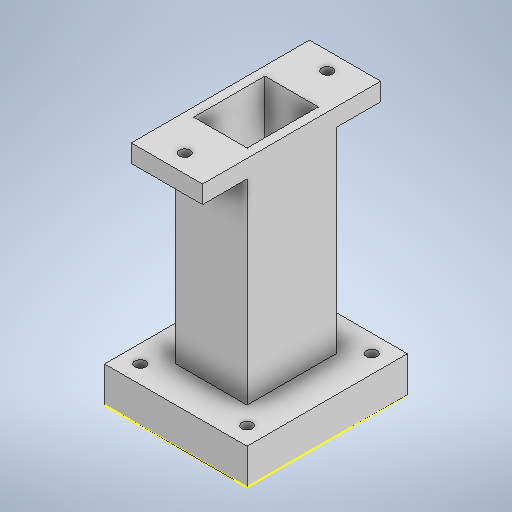
# Autodesk Inventor part: select support V3
Saved by Autodesk Inventor 2025.3 (Build 293356000, 356)
## iProperties
Created: 2026-05-01
Part Number: select support V3
Material: Generic
Document SubType Name: Modeling
Designer: kamal
Density: 1 g/cm^3
Appearance: Default
Author: kamal
## iProperties of the stored document select support V3_3DPrint.ipt
Created: 2026-05-01
Part Number: select support V3_3DPrint
Material: Generic
Document SubType Name: Modeling
Designer: kamal
Density: 1 g/cm^3
Appearance: Default
Author: kamal
Autodesk Inventor part; units mm, degrees
ref_plane "YZ Plane" through (0, 0, 0) normal (1, 0, 0) x (0, 1, 0)
ref_plane "XZ Plane" through (0, 0, 0) normal (0, 1, 0) x (-1, 0, 0)
ref_plane "XY Plane" through (0, 0, 0) normal (0, 0, 1) x (1, 0, 0)
sketch "Sketch1" plane through (0, 0, 0) normal (0, 1, 0) x (-1, 0, 0)
  line L0 (0, 0) -> (5, 0)
  line L1 (5, 0) -> (5, -10)
  line L2 (5, -10) -> (0, -10)
  line L3 (0, -10) -> (0, 0)
  line L4 (-7.5, 20) -> (12.5, 20)
  line L5 (12.5, 20) -> (12.5, -30)
  line L6 (12.5, -30) -> (-7.5, -30)
  line L7 (-7.5, -30) -> (-7.5, 20)
  line L8 (-7.5, 20) -> (12.5, -30) construction
  line L9 (12.5, 20) -> (-7.5, -30) construction
  line L10 (12.5, -17.5) -> (12.5, 7.5)
  line L11 (12.5, 7.5) -> (-7.5, 7.5)
  line L12 (-7.5, 7.5) -> (-7.5, -17.5)
  line L13 (-7.5, -17.5) -> (12.5, -17.5)
  point P0 (2.5, -5)
  point P1 (-7.5, 7.5)
  dimension "d0" = 5
  dimension "d1" = 10
  dimension "d2" = 20
  dimension "d3" = 50
  dimension "d4" = 7.5
  dimension "d5" = 20
  dimension "d6" = 7.5
  constraints: 28 end point, 6 parallel, 3 perpendicular, 2 horizontal, 2 midpoint, 3 other
  measures "d0" distance of L1.end L2.end
  measures "d1" distance of L0.end L1.end
  measures "d2" distance of L5.end L6.end
  measures "d3" distance of L4.end L5.end
  measures "d4" distance between parallel lines of L5 L1
  measures "d5" distance between parallel lines of L4 L0
  measures "d6" distance between parallel lines of L1 L10
extrude "Extrusion1" add sketch "Sketch1" along normal blind 5
extrude "Extrusion2" add sketch "Sketch1" against normal blind 55 contours L11 L5 L13 L7
sketch "Sketch2" plane through (0, -55, 0) normal (0, -1, 0) x (1, 0, 0)
  line L0 (-12.5, 7.5) -> (-12.5, -17.5) projected
  line L1 (-12.5, -17.5) -> (7.5, -17.5) projected
  line L2 (7.5, -17.5) -> (7.5, 7.5) projected
  line L3 (7.5, 7.5) -> (-12.5, 7.5) projected
  line L4 (-5, 0) -> (0, 0) projected
  line L5 (0, 0) -> (0, -10) projected
  line L6 (0, -10) -> (-5, -10) projected
  line L7 (-5, -10) -> (-5, 0) projected
  line L8 (17.5, 17.5) -> (17.5, -27.5)
  line L9 (17.5, -27.5) -> (-22.5, -27.5)
  line L10 (-22.5, -27.5) -> (-22.5, 17.5)
  line L11 (-22.5, 17.5) -> (17.5, 17.5)
  line L12 (12.5, -22.5) -> (12.5, 12.5) construction
  line L13 (12.5, 12.5) -> (-17.5, 12.5) construction
  line L14 (-17.5, 12.5) -> (-17.5, -22.5) construction
  line L15 (-17.5, -22.5) -> (12.5, -22.5) construction
  circle A0 centre (12.5, 12.5) radius 1.5
  circle A1 centre (12.5, -22.5) radius 1.5
  circle A2 centre (-17.5, 12.5) radius 1.5
  circle A3 centre (-17.5, -22.5) radius 1.5
  dimension "d11" = 10
  dimension "d12" = 5
  dimension "d13" = 3
  dimension "d14" = 3
  dimension "d15" = 3
  dimension "d16" = 3
  constraints: 16 end point, 4 centre point, 4 coincident, 6 other
  measures "d11" distance between parallel lines of L2 L8
  measures "d12" distance between parallel lines of L8 L12
  measures "d13" diameter of A0
  measures "d14" diameter of A1
  measures "d15" diameter of A2
  measures "d16" diameter of A3
extrude "Extrusion3" add sketch "Sketch2" along normal blind 10 contours L8 L9 L10 L11
sketch "Sketch3" plane through (0, 5, 0) normal (0, 1, 0) x (1, 0, 0)
  line L0 (7.5, -20) -> (7.5, 30) projected
  line L1 (7.5, 30) -> (-12.5, 30) projected
  line L2 (-12.5, 30) -> (-12.5, -20) projected
  line L3 (-12.5, -20) -> (7.5, -20) projected
  line L4 (0, 0) -> (-5, 0) projected
  line L5 (-5, 0) -> (-5, 10) projected
  line L6 (-5, 10) -> (0, 10) projected
  line L7 (0, 10) -> (0, 0) projected
  line L8 (5, 15) -> (-10, 15)
  line L9 (-10, 15) -> (-10, -5)
  line L10 (-10, -5) -> (5, -5)
  line L11 (5, -5) -> (5, 15)
  dimension "d19" = 5
  constraints: 8 end point, 3 other
  measures "d19" distance between parallel lines of L6 L8
extrude "Extrusion4" cut sketch "Sketch3" against normal through all contours L11 L10 L9 L8
sketch "Sketch4" plane through (0, -55, 0) normal (0, -1, 0) x (1, 0, 0)
  line L0 (-10, 5) -> (5, 5) projected
  line L1 (5, 5) -> (5, -15) projected
  line L2 (5, -15) -> (-10, -15) projected
  line L3 (-10, -15) -> (-10, 5) projected
  line L4 (-12.5, 7.5) -> (-12.5, -17.5) projected
  line L5 (-12.5, -17.5) -> (7.5, -17.5) projected
  line L6 (7.5, -17.5) -> (7.5, 7.5) projected
  line L7 (7.5, 7.5) -> (-12.5, 7.5) projected
  point P0 (0, 0)
extrude "Extrusion5" add sketch "Sketch4" along normal blind 10
sketch "Sketch5" plane through (0, 5, 0) normal (0, 1, 0) x (1, 0, 0)
  line L0 (5, -5) -> (-10, -5) projected
  line L1 (-10, -5) -> (-10, 15) projected
  line L2 (-10, 15) -> (5, 15) projected
  line L3 (5, 15) -> (5, -5) projected
  line L4 (7.5, -20) -> (7.5, 30) projected
  line L5 (7.5, 30) -> (-12.5, 30) projected
  line L6 (-12.5, 30) -> (-12.5, -20) projected
  line L7 (-12.5, -20) -> (7.5, -20) projected
  circle A0 centre (-2.5, -15) radius 1.5
  circle A1 centre (-2.5, 25) radius 1.5
  point P0 (0, 0)
  dimension "d24" = 3
  dimension "d25" = 3
  dimension "d26" = 10
  dimension "d27" = 10
  dimension "d28" = 10
  dimension "d29" = 10
  constraints: 2 centre point
  measures "d24" diameter of A0
  measures "d25" diameter of A1
  measures "d26" distance from line of L0 A0.centre
  measures "d27" distance from line of L2 A1.centre
  measures "d28" distance from line of L6 A0.centre
  measures "d29" distance from line of L6 A1.centre
extrude "Extrusion6" cut sketch "Sketch5" against normal blind 10 contours A0 | A1
sketch "Sketch6" plane through (0, -65, 0) normal (0, -1, 0) x (1, 0, 0)
  line L0 (-10, 5) -> (5, 5) projected
  line L1 (5, 5) -> (5, -15) projected
  line L2 (5, -15) -> (-10, -15) projected
  line L3 (-10, -15) -> (-10, 5) projected
  line L4 (-22.5, 17.5) -> (-22.5, -27.5) projected
  line L5 (-22.5, -27.5) -> (17.5, -27.5) projected
  line L6 (17.5, -27.5) -> (17.5, 17.5) projected
  line L7 (17.5, 17.5) -> (-22.5, 17.5) projected
  circle A0 centre (12.5, 12.5) radius 1.5 projected
  circle A1 centre (12.5, -22.5) radius 1.5 projected
  circle A2 centre (-17.5, 12.5) radius 1.5 projected
  circle A3 centre (-17.5, -22.5) radius 1.5 projected
  point P0 (0, 0)
body "Solid1"
